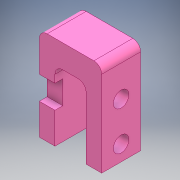
# Autodesk Inventor part: crochet
Saved by Autodesk Inventor 2017 (Build 210142000, 142)
## iProperties
Created: 2017-04-13
Part Number: crochet
Material: Generic
Document SubType Name: Modeling
Designer: franc
Density: 1 g/cm^3
Appearance: Default
Author: franc
Autodesk Inventor part; units mm, degrees
ref_plane "YZ Plane" through (0, 0, 0) normal (1, 0, 0) x (0, 1, 0)
ref_plane "XZ Plane" through (0, 0, 0) normal (0, 1, 0) x (-1, 0, 0)
ref_plane "XY Plane" through (0, 0, 0) normal (0, 0, 1) x (1, 0, 0)
sketch "Sketch1" plane through (0, 0, 0) normal (0, 1, 0) x (-1, 0, 0)
  line L0 (-4.0561, -5.7426) -> (-4.0561, 5.2574)
  line L1 (-3.0561, 6.2574) -> (2.9439, 6.2574)
  line L2 (3.9439, 5.2574) -> (3.9439, -5.7426)
  line L3 (3.9439, -5.7426) -> (1.9439, -5.7426)
  line L4 (1.9439, -5.7426) -> (1.9439, 2.2574)
  line L5 (0.9439, 3.2574) -> (-1.0561, 3.2574)
  line L6 (-2.0561, 2.2574) -> (-2.0561, -5.7426)
  line L7 (-2.0561, -5.7426) -> (-4.0561, -5.7426)
  arc A0 (-1.0561, 3.2574) -> (-2.0561, 2.2574) centre (-1.0561, 2.2574) ccw
  arc A1 (1.9439, 2.2574) -> (0.9439, 3.2574) centre (0.9439, 2.2574) ccw
  arc A2 (-3.0561, 6.2574) -> (-4.0561, 5.2574) centre (-3.0561, 5.2574) ccw
  arc A3 (3.9439, 5.2574) -> (2.9439, 6.2574) centre (2.9439, 5.2574) ccw
  point P0 (0, 0)
  point P1 (-4.0561, 6.2574)
  point P2 (3.9439, 6.2574)
  point P3 (1.9439, 3.2574)
  point P4 (-2.0561, 3.2574)
  dimension "d0" = 12
  dimension "d1" = 2
  dimension "d2" = 2
  dimension "d3" = 8
  dimension "d4" = 3
  dimension "d20" = 1
  constraints: 16 end point, 9 point on line, 8 point on circle, 8 tangent, 7 perpendicular, 4 centre point, 3 equal radius, 1 vertical
  measures "d0" distance of L0.start point (-4.056, 6.257)
  measures "d1" distance of L6.end L0.start
  measures "d2" distance of L2.end L3.end
  measures "d3" distance of point (-4.056, 6.257) point (3.944, 6.257)
  measures "d4" distance between parallel lines of L1 L5
  measures "d20" radius of A0
extrude "Extrusion1" add sketch "Sketch1" along normal blind 5
sketch "Sketch2" plane through (4.0561, 0, 6.2574) normal (1, 0, 0) x (0, 0, -1)
  circle A0 centre (10, 2.5) radius 1
  circle A1 centre (5, 2.5) radius 1
  line L0 (12, 0) -> (12, 5) projected
  line L1 (1, 5) -> (12, 5) projected
  point P0 (6.2574, 0)
  point P1 (0, 5)
  dimension "d7" = 2
  dimension "d8" = 2
  dimension "d9" = 2
  dimension "d10" = 2.5
  dimension "d11" = 2.5
  dimension "d12" = 5
  constraints: 2 centre point
  measures "d7" diameter of A0
  measures "d8" diameter of A1
  measures "d9" distance from line of L0 A0.centre
  measures "d10" distance from line of L1 A0.centre
  measures "d11" distance from line of L1 A1.centre
  measures "d12" distance of A0.centre A1.centre
extrude "Extrusion2" cut sketch "Sketch2" against normal up to surface (2 mm away)
sketch "Sketch3" plane through (-3.9439, 0, -5.7426) normal (-1, 0, 0) x (0, 0, 1)
  line L0 (7, 0.0877) -> (7, 1)
  line L1 (7, 1) -> (4, 1)
  line L2 (4, 1) -> (4, 0)
  line L3 (0, 0) -> (11, 0) projected
  line L4 (11, 5) -> (0, 5) projected
  line L5 (7, 5) -> (7, 4)
  line L6 (7, 4) -> (4, 4)
  line L7 (4, 4) -> (4, 5)
  line L8 (7, 0.0877) -> (7, 0)
  line L9 (0, 0) -> (0, 5) projected
  point P0 (5.7426, 0)
  point P1 (12, 0)
  point P2 (12, 5)
  dimension "d15" = 1
  dimension "d16" = 1
  dimension "d17" = 3
  dimension "d21" = 4
  constraints: 14 end point, 9 point on line, 3 perpendicular, 1 vertical
  measures "d15" distance of L1.end L2.end
  measures "d16" distance of L6.end L7.end
  measures "d17" distance of L5.end L6.end
  measures "d21" distance between parallel lines of L9 L7
extrude "Extrusion3" cut sketch "Sketch3" against normal up to next
body "Solid1"
